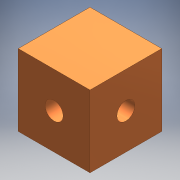
# Autodesk Inventor part: 垂直ブロック 樹脂 10
Saved by Autodesk Inventor 2016 (Build 200138000, 138)
## iProperties
Created: 2019-03-21
Part Number: 垂直ブロック 樹脂 10
Material: PPS プラスチック
Document SubType Name: Modeling
Designer: mozar
Density: 1.637 g/cm^3
Appearance: 滑らか - 濃い茶
Author: mozar
Autodesk Inventor part; units mm, degrees
ref_plane "YZ Plane" through (0, 0, 0) normal (1, 0, 0) x (0, 1, 0)
ref_plane "XZ Plane" through (0, 0, 0) normal (0, 1, 0) x (-1, 0, 0)
ref_plane "XY Plane" through (0, 0, 0) normal (0, 0, 1) x (1, 0, 0)
sketch "スケッチ1" plane through (0, 0, 0) normal (0, 0, 1) x (1, 0, 0)
  line L0 (0, 0) -> (10, 0)
  line L1 (10, 0) -> (10, -10)
  line L2 (10, -10) -> (0, -10)
  line L3 (0, -10) -> (0, 0)
  line L4 (0, -5) -> (10, -5)
  line L5 (5, 0) -> (5, -10)
  dimension "d0" = 10
  dimension "d1" = 10
  constraints: 12 end point, 4 midpoint, 2 parallel, 1 horizontal, 1 perpendicular
  measures "d0" distance of L1.end L2.end
  measures "d1" distance of L0.end L1.end
extrude "押し出し1" add sketch "スケッチ1" along normal blind 10
sketch "スケッチ2" plane through (10, -10, 0) normal (1, 0, 0) x (0, 0, -1)
  line L0 (-10, 10) -> (0, 10) projected
  line L1 (0, 10) -> (0, 0) projected
  line L2 (0, 0) -> (-10, 0) projected
  line L3 (-10, 0) -> (-10, 10) projected
  line L4 (-10, 10) -> (0, 0)
  line L5 (0, 10) -> (0, 0) projected
  line L6 (-10, 0) -> (0, 10)
  point P0 (-5, 5)
  constraints: 4 end point, 1 midpoint
hole "穴1" at (10, -5, 5) direction (-1, 0, 0) diameter 2.5 end through all
sketch "スケッチ3" plane through (0, 0, 0) normal (0, 1, 0) x (1, 0, 0)
  line L0 (10, 0) -> (10, -10) projected
  line L1 (10, -10) -> (0, -10) projected
  line L2 (0, -10) -> (0, 0) projected
  line L3 (0, 0) -> (10, 0) projected
  line L4 (0, -10) -> (10, 0)
  line L5 (10, 0) -> (10, -10) projected
  line L6 (0, 0) -> (10, 0) projected
  line L7 (10, -10) -> (0, 0)
  point P0 (5, -5)
  constraints: 4 end point, 1 midpoint, 1 perpendicular
hole "穴2" at (5, 0, 5) direction (0, -1, 0) diameter 2.5 end through all
